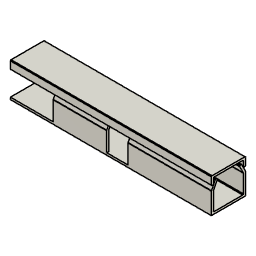
colour_detection_mechanism_conduit (Autodesk Fusion 360 design; units mm, degrees)
Autodesk Fusion 360 part; units mm, degrees
sketch "16 mm x 16 mm conduit piping shape" plane through (0, 0, 0) normal (1, 0, 0) x (0, 1, 0)
  line L0 (0, 0) -> (16, 0)
  line L1 (16, 0) -> (16, 10)
  line L2 (16, 10) -> (14, 13.9)
  line L3 (14, 13.9) -> (13.1102, 13.4437)
  line L4 (13.1102, 13.4437) -> (15, 9.7585)
  line L5 (15, 9.7585) -> (15, 1)
  line L6 (15, 1) -> (1, 1)
  line L7 (1, 1) -> (1, 9.7585)
  line L8 (1, 9.7585) -> (2.8898, 13.4437)
  line L9 (2.8898, 13.4437) -> (2, 13.9)
  line L10 (2, 13.9) -> (0, 10)
  line L11 (0, 10) -> (0, 0)
  line L12 (0, 16) -> (16, 16)
  line L13 (0, 16) -> (0, 12)
  line L14 (0, 12) -> (1, 12)
  line L15 (1, 12) -> (1, 15)
  line L16 (1, 15) -> (15, 15)
  line L17 (15, 15) -> (15, 12)
  line L18 (15, 12) -> (16, 12)
  line L19 (16, 12) -> (16, 16)
  dimension "d1" = 1
  dimension "d2" = 16
  dimension "d3" = 1
  dimension "d4" = 1
  dimension "d7" = 10
  dimension "d8" = 10
  dimension "d9" = 16
  dimension "d10" = 1
  dimension "d11" = 1
  dimension "d12" = 1
  dimension "d13" = 4
  dimension "d14" = 4
  dimension "d15" = 16
  dimension "d16" = 2
  dimension "d17" = 2
  dimension "d18" = 1
  dimension "d19" = 1
  constraint coincident L0.start L11.end
  constraint horizontal L0
  constraint perpendicular L0 L1
  constraint perpendicular L2 L3
  constraint parallel L1 L5
  constraint perpendicular L5 L6
  constraint perpendicular L6 L7
  constraint perpendicular L0 L11
  constraint horizontal L12
  constraint perpendicular L12 L13
  constraint perpendicular L13 L14
  constraint perpendicular L14 L15
  constraint perpendicular L15 L16
  constraint perpendicular L16 L17
  constraint perpendicular L17 L18
  constraint perpendicular L12 L19
  constraint parallel L8 L10
  constraint parallel L2 L4
  constraint perpendicular L9 L10
  measures "d1" distance of L0 L6
  measures "d2" distance of L1 L11
  measures "d3" distance of L7 L11
  measures "d4" distance of L1 L5
  measures "d7" distance of L0.end L1.end
  measures "d8" distance of L10.end L0.start
  measures "d9" distance of L0 L12
  measures "d10" distance of L12 L16
  measures "d11" distance of L17 L19
  measures "d12" distance of L13 L15
  measures "d13" distance of L12.end L18.end
  measures "d14" distance of L12.start L13.end
  measures "d15" distance of L12.start L12.end
  measures "d16" horizontal distance of L1.end L2.end
  measures "d17" horizontal distance of L9.end L10.end
  measures "d18" distance of L2.end L3.end
  measures "d19" distance of L8.end L9.end
extrude "Extrude1" add sketch "16 mm x 16 mm conduit piping shape" along normal blind 94 makes body 1 at (31.3333, 5.3333, 16) makes body 2 at (31.3333, 5.3333, 0)
fillet "Fillet1" radius 0.3 18 edges at (47, 0, 16) (47, 16, 16) (47, 16, 12) (47, 0, 12) (47, 1, 12) (47, 15, 12) (47, 1, 15) (47, 15, 15) (47, 0, 10) (47, 16, 10) (47, 14, 13.9) (47, 13.1102, 13.4437) (47, 2, 13.9) (47, 2.8898, 13.4437) (47, 15, 1) (47, 1, 1) (47, 1, 9.7585) (47, 15, 9.7585) on bodies 1 2
sketch "Sketch2" plane through (0, 0, 0) normal (0, -1, 0) x (1, 0, 0)
  line L0 (94, 9.9276) -> (0, 9.9276)
  line L1 (0, 9.9276) -> (0, 0)
  line L2 (0, 0) -> (94, 0)
  line L3 (94, 0) -> (94, 9.9276)
  line L4 (0, 15) -> (20, 15)
  line L5 (20, 15) -> (20, 1)
  line L6 (20, 1) -> (0, 1)
  line L7 (0, 1) -> (0, 15)
  line L8 (45, 15) -> (55, 15)
  line L9 (55, 15) -> (55, 1)
  line L10 (55, 1) -> (45, 1)
  line L11 (45, 1) -> (45, 15)
  dimension "d25" = 20
  dimension "d26" = 1
  dimension "d27" = 25
  dimension "d28" = 10
  dimension "d29" = 1
  constraint horizontal L4
  constraint vertical L5
  constraint horizontal L6
  constraint vertical L7
  constraint horizontal L8
  constraint vertical L9
  constraint horizontal L10
  constraint vertical L11
  measures "d25" distance of L5 L7
  measures "d26" distance of L2 L6
  measures "d27" distance of L5 L11
  measures "d28" distance of L9.end L10.end
  measures "d29" distance of L2 L10
extrude "Extrude2" cut sketch "Sketch2" against normal blind 3 contours L0 L9 L10 L11 | L0 L8 L9 L11 | L0 L1 L5 L6 L7 | L0 L4 L5 L7 bodies 2
sketch "Sketch3" plane through (0, 16, 0) normal (0, 1, 0) x (-1, 0, 0)
  line L0 (0, 9.9276) -> (-94, 9.9276)
  line L1 (-94, 9.9276) -> (-94, 0)
  line L2 (-94, 0) -> (0, 0)
  line L3 (0, 0) -> (0, 9.9276)
  line L4 (0, 15) -> (-20, 15)
  line L5 (-20, 15) -> (-20, 1)
  line L6 (-20, 1) -> (0, 1)
  line L7 (0, 1) -> (0, 15)
  dimension "d32" = 20
  dimension "d33" = 1
  constraint horizontal L4
  constraint vertical L5
  constraint horizontal L6
  constraint vertical L7
  measures "d32" distance of L4.start L4.end
  measures "d33" distance of L2 L6
extrude "Extrude3" cut sketch "Sketch3" against normal blind 3 contours L0 L3 L5 L6 L7 | L0 L4 L5 L7 bodies 2
sketch "Sketch4" plane through (0, 16, 0) normal (0, 1, 0) x (-1, 0, 0)
  line L0 (-20, 1) -> (-20, 9.9276)
  line L1 (-20, 9.9276) -> (-94, 9.9276)
  line L2 (-94, 9.9276) -> (-94, 0)
  line L3 (-94, 0) -> (0, 0)
  line L4 (0, 0) -> (0, 1)
  line L5 (0, 1) -> (-20, 1)
  line L6 (-45, 1) -> (-45, 15)
  line L7 (-45, 15) -> (-55, 15)
  line L8 (-55, 15) -> (-55, 1)
  line L9 (-55, 1) -> (-45, 1)
  line L10 (-55, 1) -> (-40, 1)
  line L11 (-40, 1) -> (-40, 15)
  line L12 (-40, 15) -> (-55, 15)
  line L13 (-55, 15) -> (-55, 1)
  dimension "d36" = 15
  constraint horizontal L10
  constraint vertical L11
  constraint horizontal L12
  constraint vertical L13
  constraint coincident L8.end L9.start
  constraint collinear L7 L12
  measures "d36" distance of L8.end L10.end
extrude "Extrude4" cut sketch "Sketch4" against normal blind 3 contours L1 L6 L10 L11 | L1 L6 L11 L12 | L1 L6 L8 L9 L10 L13 | L1 L6 L7 L8 L12 L13 bodies 2
equation "d1 = conduitThickness"
equation "d2 = conduitWidth"
equation "d3 = conduitThickness"
equation "d4 = conduitThickness"
equation "conduitThickness = 1 mm" comment "Thickness of the PVC conduit piping"
equation "conduitWidth = 16 mm" comment "Size of the outer dimensions of the conduit piping"
equation "d9 = conduitWidth"
equation "d10 = conduitThickness"
equation "d11 = conduitThickness"
equation "d12 = conduitThickness"
named bodies: "sorting mechanism conduit top", "sorting mechanism conduit bottom"
